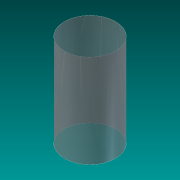
# Autodesk Inventor part: 円柱
Saved by Autodesk Inventor 2016 (Build 200138000, 138)
## iProperties
Created: 2016-05-14
Part Number: 円柱
Material: 一般
Document SubType Name: Modeling
Designer: hiroaki
Appearance: クリア
Surface Area: 9785.79 cm^2
Volume: 48.9197 cm^3
Author: hiroaki
Autodesk Inventor part; units mm, degrees
ref_plane "YZ Plane" through (0, 0, 0) normal (1, 0, 0) x (0, 1, 0)
ref_plane "XZ Plane" through (0, 0, 0) normal (0, 1, 0) x (-1, 0, 0)
ref_plane "XY Plane" through (0, 0, 0) normal (0, 0, 1) x (1, 0, 0)
sketch "スケッチ1" plane through (0, 0, 0) normal (0, 0, 1) x (1, 0, 0)
  circle A0 centre (0, 0) radius 156.75
  circle A1 centre (0, 0) radius 156.85
  dimension "d0" = 313.5
  dimension "d1" = 0.1
  constraints: 2 centre point, 2 coincident
  measures "d0" diameter of A0
  measures "d1" radial gap between concentric circles of A1 A0
extrude "押し出し1" add sketch "スケッチ1" along normal blind 570
equation "\"d0\" = 0.55 * H_top"
equation "\"d2\" = H_top"
equation "\"H_head\" = 28.5"
equation "\"H_leg\" = 199.5"
equation "\"H_top\" = 570"
equation "\"足の面積\" = 12720.125"
equation "\"現在の面積\" = 11560"
equation "\"足_短辺\" = 68"
equation "\"円柱\" = 313.5"
equation "\"胴体中心から手先\" = 342"
equation "\"H_leg_1\" = 186.2"
equation "\"H_leg_MAX\" = 399"
equation "\"H_head_1\" = 26.6"
equation "\"H_head_MAX\" = 142.5"
